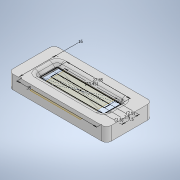
# Autodesk Inventor part: Capping_Cover
Saved by Autodesk Inventor 2022 (Build 260153000, 153)
## iProperties
Created: 2024-04-10
Part Number: Capping_Cover
Material: Generic
Document SubType Name: Modeling
Designer: Gotham City
Density: 1 g/cm^3
Appearance: Default
Author: Gotham City
Autodesk Inventor part; units mm, degrees
ref_plane "YZ Plane" through (0, 0, 0) normal (1, 0, 0) x (0, 1, 0)
ref_plane "XZ Plane" through (0, 0, 0) normal (0, 1, 0) x (-1, 0, 0)
ref_plane "XY Plane" through (0, 0, 0) normal (0, 0, 1) x (1, 0, 0)
sketch "Sketch1" plane through (0, 0, 0) normal (0, 1, 0) x (-1, 0, 0)
  line L0 (13.925, -3.75) -> (-13.925, -3.75)
  line L1 (-13.925, -3.75) -> (-13.925, 3.75)
  line L2 (-13.925, 3.75) -> (13.925, 3.75)
  line L3 (13.925, 3.75) -> (13.925, -3.75)
  line L4 (13.925, -3.75) -> (-13.925, 3.75) construction
  line L5 (-13.925, -3.75) -> (13.925, 3.75) construction
  line L6 (11.725, -1.25) -> (-11.725, -1.25)
  line L7 (-11.725, -1.25) -> (-11.725, 1.25)
  line L8 (-11.725, 1.25) -> (11.725, 1.25)
  line L9 (11.725, 1.25) -> (11.725, -1.25)
  line L10 (11.725, -1.25) -> (-11.725, 1.25) construction
  line L11 (-11.725, -1.25) -> (11.725, 1.25) construction
  line L12 (11.725, -1.25) -> (11.725, -3.75) construction
  line L13 (11.725, 1.25) -> (11.725, 3.75) construction
  line L14 (11.725, -1.25) -> (13.925, -1.25) construction
  line L15 (-11.725, -1.25) -> (-13.925, -1.25) construction
  point P0 (0, 0)
  point P1 (0, 0)
  point P2 (0, 0)
  point P3 (0, 0)
  dimension "d0" = 27.85
  dimension "d1" = 7.5
  dimension "d2" = 2.5
  dimension "d3" = 2.5
  dimension "d4" = 2.5
  dimension "d5" = 2.2
  dimension "d6" = 23.45
  constraints: 32 end point, 6 point on line, 5 midpoint, 4 parallel, 4 perpendicular, 2 collinear, 2 horizontal, 1 coincident
  measures "d0" distance of L0.start L0.end
  measures "d1" distance of L0.end L1.end
  measures "d2" distance between parallel lines of L0 L6
  measures "d3" distance between parallel lines of L2 L8
  measures "d4" distance of L6.end L7.end
  measures "d5" distance of L6.end L15.end
  measures "d6" distance of L6.start L6.end
sketch "Sketch2" plane through (0, 0, 0) normal (0, 1, 0) x (-1, 0, 0)
  line L0 (17.5, 8) -> (-17.5, 8)
  line L1 (-17.5, 8) -> (-17.5, -8)
  line L2 (-17.5, -8) -> (17.5, -8)
  line L3 (17.5, -8) -> (17.5, 8)
  line L4 (17.5, 8) -> (-17.5, -8) construction
  point P0 (0, 0)
  point P1 (0, 0)
  dimension "d7" = 35
  dimension "d8" = 16
  constraints: 10 end point, 2 parallel, 1 coincident, 1 horizontal, 1 midpoint, 1 perpendicular
  measures "d7" distance of L0.start L0.end
  measures "d8" distance of L2.end L0.start
ref_plane "Work Plane1" through (0, 0, 0) normal (0, 1, 0) x (1, 0, 0)
sketch "Sketch7" plane through (0, 0, 0) normal (0, 1, 0) x (1, 0, 0)
  line L0 (-21.5, -10) -> (21.5, -10)
  line L1 (21.5, -10) -> (21.5, 10)
  line L2 (21.5, 10) -> (-21.5, 10)
  line L3 (-21.5, 10) -> (-21.5, -10)
  line L4 (-41.9153, 0) -> (40.6847, 0) construction
  line L5 (0, 14.4923) -> (0, -13.5077) construction
  line L6 (-17.5, 8) -> (-17.5, -7.5077) construction
  line L7 (16.9462, 8) -> (-17.5, 8) construction
  line L8 (17.5, 8) -> (-17.5, 8) construction
  line L9 (-17.5, 8) -> (-17.5, -8) construction
  line L10 (0, 20.0923) -> (0, -19.1077) construction
  line L11 (57.2047, 0) -> (-58.4353, 0) construction
  point P0 (0, 0)
  dimension "d20" = 4
  dimension "d21" = 2
  dimension "d51" = 0
  dimension "d52" = 0
  constraints: 16 end point, 2 parallel, 1 horizontal, 1 perpendicular, 2 other
  measures "d20" distance between parallel lines of L3 L6
  measures "d21" distance between parallel lines of L2 L7
  measures "d51" distance between parallel lines of L11 L4
  measures "d52" distance between parallel lines of L10 L5
extrude "Extrusion4" add sketch "Sketch7" along normal blind 1.5
extrude "Extrusion5" add sketch "Sketch7" against normal blind 4
extrude "Extrusion6" cut sketch "Sketch2" against normal through all
extrude "Extrusion7" cut sketch "Sketch1" along normal through all contours L0 L1 L2 L3 | L6 L7 L8 L9
thicken "Thicken1" operation add thickness 0.4 both sides no extend neighbours yes toward (0, 0, 1) faces at (-4.6417, 0.5, 3.75) (13.925, 0.5, 1.25) (-13.925, 0.5, -1.25) (4.6417, 0.5, -3.75)
fillet "Fillet6" radius 1 4 edges at (14.325, 0.75, 4.15) (-14.325, 0.75, 4.15) (-14.325, 0.75, -4.15) (14.325, 0.75, -4.15)
chamfer "Chamfer2" distance 1.5 angle 45 8 edges at (14.325, 1.5, 0) (14.0321, 1.5, 3.8571) (0, 1.5, 4.15) (-14.0321, 1.5, 3.8571) (-14.325, 1.5, 0) (-14.0321, 1.5, -3.8571) (0, 1.5, -4.15) (14.0321, 1.5, -3.8571)
fillet "Fillet7" radius 2 8 edges at (15.0927, 1.5, 4.9177) (15.8249, 1.5, 0) (15.0927, 1.5, -4.9177) (0, 1.5, -5.6499) (-15.0927, 1.5, -4.9177) (-15.8249, 1.5, 0) (-15.0927, 1.5, 4.9177) (0, 1.5, 5.6499)
sketch "Sketch8" plane through (-29.5, -4, -10) normal (0, -1, 0) x (1, 0, 0)
  circle A0 centre (53, 10) radius 5
  line L0 (47, 18) -> (47, 2) projected
  line L1 (51, 0) -> (51, 20) projected
  point P0 (29.5, 10)
  point P1 (47, 10)
  point P2 (51, 10)
  dimension "d46" = 10
  dimension "d49" = 23.5
  constraints: 2 midpoint, 1 centre point, 1 horizontal alignment
  measures "d46" diameter of A0
  measures "d49" distance of A0.centre point (29.5, 10)
extrude "Extrusion9" [suppressed]
mirror "Mirror1" [suppressed]
fillet "Fillet8" radius 2 4 edges at (21.5, -1.25, 10) (21.5, -1.25, -10) (-21.5, -1.25, -10) (-21.5, -1.25, 10)
thicken "Thicken3" operation add thickness 0.05 both sides no extend neighbours yes toward (0, 0, 1) faces at (-5.8333, -2.6667, 8) (-17.5, -1.3333, -2.6667) (17.5, -2.6667, 2.6667) (5.8333, -1.3333, -8)
thicken "Thicken4" operation add thickness 0.5 both sides no extend neighbours yes toward (0, -1, 0) faces at (-5.85, -4, -9.35)
body "Solid1"
body "Solid2"
